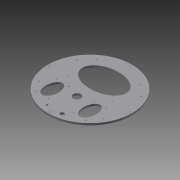
# Autodesk Inventor part: Base_Acryllic
Saved by Autodesk Inventor 2015 SP1 (Build 190203100, 203)
## iProperties
Created: 2016-03-29
Part Number: Base_Acryllic
Material: Generic
Document SubType Name: Modeling
Designer: Ethan
Density: 1 g/cm^3
Appearance: Default
Author: Ethan
Autodesk Inventor part; units mm, degrees
ref_plane "YZ Plane" through (0, 0, 0) normal (1, 0, 0) x (0, 1, 0)
ref_plane "XZ Plane" through (0, 0, 0) normal (0, 1, 0) x (-1, 0, 0)
ref_plane "XY Plane" through (0, 0, 0) normal (0, 0, 1) x (1, 0, 0)
sketch "Sketch1" plane through (0, 0, 0) normal (0, 1, 0) x (-1, 0, 0)
  circle A0 centre (0, 0) radius 139.7
  circle A1 centre (107.2204, 62.9369) radius 1.5875
  circle A2 centre (-107.2204, 62.9369) radius 1.5875
  circle A3 centre (107.2204, -62.9369) radius 1.5875
  circle A4 centre (-107.2204, -62.9369) radius 1.5875
  circle A5 centre (73.2444, -95.6484) radius 1.5875
  circle A6 centre (73.2444, -0.3984) radius 1.5875
  circle A7 centre (-73.025, -0.3984) radius 1.5875
  circle A8 centre (-72.8056, -95.6484) radius 1.5875
  ellipse E0 centre (0.4389, -48.0234) end of major axis (-72.5861, -48.0234) minor radius 47.625
  circle A9 centre (0, 133.35) radius 1.5875
  circle A10 centre (-133.35, 0) radius 1.5875
  circle A11 centre (0, -133.35) radius 1.5875
  circle A12 centre (133.35, 0) radius 1.5875
  circle A13 centre (-25.4, 117.8713) radius 6.35
  circle A14 centre (25.4, 117.8713) radius 3.175
  circle A15 centre (-83.3566, 29.2053) radius 1.5875
  circle A16 centre (-41.7006, 29.2053) radius 1.5875
  circle A17 centre (-41.7006, 96.5153) radius 1.5875
  circle A18 centre (-83.3566, 96.5153) radius 1.5875
  ellipse E1 centre (-62.5286, 62.8603) end of major axis (-62.5286, 29.2053) minor radius 20.828
  circle A19 centre (6.25, 127) radius 1.1303
  circle A20 centre (-6.25, 127) radius 1.1303
  circle A21 centre (-127, -6.25) radius 1.1303
  circle A22 centre (-127, 6.25) radius 1.1303
  circle A23 centre (6.25, -127) radius 1.1303
  circle A24 centre (-6.25, -127) radius 1.1303
  circle A25 centre (127, 6.25) radius 1.1303
  circle A26 centre (127, -6.25) radius 1.1303
  circle A27 centre (0, 42.9864) radius 12.7
  circle A28 centre (41.7006, 29.2053) radius 1.5875
  circle A29 centre (83.3566, 29.2053) radius 1.5875
  ellipse E2 centre (62.5286, 62.8603) end of major axis (62.5286, 29.2053) minor radius 20.828
  circle A30 centre (41.7006, 96.5153) radius 1.5875
  circle A31 centre (83.3566, 96.5153) radius 1.5875
  dimension "d0" = 279.4
  dimension "d60" = 3.175
  dimension "d92" = 3.175
  dimension "d93" = 3.175
  dimension "d94" = 3.175
  dimension "d95" = 3.175
  dimension "d97" = 3.175
  dimension "d100" = 360
  dimension "d102" = 12.7
  dimension "d103" = 6.35
  dimension "d118" = 2.2606
  dimension "d121" = 50.8
  dimension "d122" = 25.4
  dimension "d123" = 25.4
  dimension "d125" = 73.025
  dimension "d126" = 146.05
  constraints: 32 centre point, 11 coincident, 15 other
  measures "d0" diameter of A0
  measures "d60" diameter of A1
  measures "d92" diameter of A5
  measures "d93" diameter of A6
  measures "d94" diameter of A7
  measures "d95" diameter of A8
  measures "d97" diameter of A9
  measures "d102" diameter of A13
  measures "d103" diameter of A14
  measures "d118" diameter of A19
  measures "d121" distance of A14.centre A13.centre
  measures "d122" horizontal distance of A9.centre A13.centre
  measures "d123" diameter of A27
  measures "d125" horizontal distance of A27.centre A7.centre
  measures "d126" distance of A5.centre A8.centre
extrude "Extrusion9" add sketch "Sketch1" along normal blind 6.35
body "Solid7"
